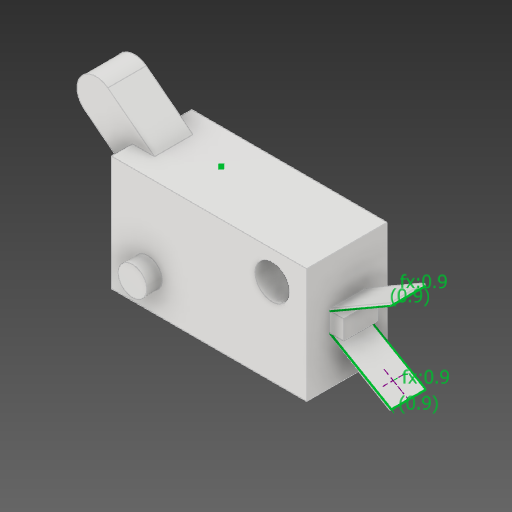
# Autodesk Inventor part: LimitSwitch
Saved by Autodesk Inventor 2019 (Build 230136000, 136)
## iProperties
Created: 2019-04-29
Part Number: LimitSwitch
Material: ABS Plastic
Document SubType Name: Modeling
Designer: skylercleland
Density: 1.06 g/cm^3
Appearance: Smooth - White
Mass: 0.281544 g
Surface Area: 3.43625 cm^2
Volume: 0.265608 cm^3
Name: Limit Switch
Author: skylercleland
Autodesk Inventor part; units mm, degrees
ref_plane "YZ Plane" through (0, 0, 0) normal (1, 0, 0) x (0, 1, 0)
ref_plane "XZ Plane" through (0, 0, 0) normal (0, 1, 0) x (-1, 0, 0)
ref_plane "XY Plane" through (0, 0, 0) normal (0, 0, 1) x (1, 0, 0)
sketch "Sketch1" plane through (0, 0, 0) normal (0, 0, 1) x (1, 0, 0)
  line L0 (0, 0) -> (10.2, 0)
  line L1 (10.2, 0) -> (10.2, 6)
  line L2 (10.2, 6) -> (0, 6)
  line L3 (0, 6) -> (0, 0)
  circle A0 centre (8.4, 4.5) radius 0.9
  line L4 (10.2, 3.5) -> (10.9353, 3.5)
  line L5 (10.9353, 3.5) -> (10.9353, 2.5)
  line L6 (10.9353, 2.5) -> (10.2, 2.5)
  line L7 (10.2, 2.5) -> (10.2, 3.5)
  line L8 (10.2, 3.5) -> (10.15, 3.5866)
  line L9 (10.15, 3.5866) -> (13.35, 5.4341)
  line L10 (13.35, 5.4341) -> (13.4, 5.3475)
  line L11 (13.4, 5.3475) -> (10.2, 3.5)
  line L12 (10.2, 2.5) -> (10.15, 2.4134)
  line L13 (10.15, 2.4134) -> (13.35, 0.5659)
  line L14 (13.35, 0.5659) -> (13.4, 0.6525)
  line L15 (13.4, 0.6525) -> (10.2, 2.5)
  circle A1 centre (1.9, 1.7) radius 0.75
  line L16 (0, 4.3634) -> (-2.5124, 6.3094)
  line L17 (-2.5124, 6.3094) -> (-1.2876, 7.8906)
  line L18 (-1.2876, 7.8906) -> (1.1531, 6)
  arc A2 (-1.2876, 7.8906) -> (-2.5124, 6.3094) centre (-1.9, 7.1) ccw
  point P0 (10.9353, 3)
  point P1 (10.2, 3)
  dimension "d0" = 10.2
  dimension "d1" = 6
  dimension "d2" = 1.8
  dimension "d3" = 1.5
  dimension "d4" = 1.8
  dimension "d5" = 2.8
  dimension "d6" = 6.5
  dimension "d7" = 1.5
  dimension "d8" = 0.1
  dimension "d9" = 0.1
  dimension "d10" = 2.1
  dimension "d11" = 13.1
  dimension "d12" = 30
  dimension "d13" = 30
  dimension "d15" = 1
  dimension "d16" = 5
  dimension "d17" = 2
  constraints: 38 end point, 9 parallel, 5 perpendicular, 3 centre point, 3 midpoint, 3 point on line, 2 horizontal, 2 point on circle, 1 horizontal alignment, 1 vertical alignment
  measures "d0" distance of L2.end L1.end
  measures "d1" distance of L1.end L0.end
  measures "d2" distance from line of L1 A0.centre
  measures "d3" distance from line of L2 A0.centre
  measures "d4" diameter of A0
  measures "d5" vertical distance of A0.centre A1.centre
  measures "d6" horizontal distance of A0.centre A1.centre
  measures "d7" diameter of A1
  measures "d8" distance between parallel lines of L15 L13
  measures "d9" distance between parallel lines of L9 L11
  measures "d12" angle of L15 L6
  measures "d13" angle of L4 L11
  measures "d15" distance between parallel lines of L6 L4
  measures "d16" horizontal distance of A0.centre L10.end
  measures "d17" distance between parallel lines of L16 L18
extrude "Extrusion1" add sketch "Sketch1" along normal mid plane 4.2 contours L3 L2 L1 L9 L8 L12 L13 L0 | L13 L12 L1 | L8 L9 L1
extrude "Extrusion2" add sketch "Sketch1" along normal mid plane 1.8 contours L13 L12 L1 | L1 L15 L14 L13 | L1 L4 L5 L6 | L8 L9 L1 | L1 L9 L10 L11
extrude "Extrusion3" add sketch "Sketch1" along normal mid plane 5.8 contours A1
extrude "Extrusion4" add sketch "Sketch1" along normal mid plane 2 contours L16 L17 L18 L2 L3 | A2 L17
sketch "Sketch2" plane through (10.2, 2.5, 0.9) normal (0.5, 0.866, 0) x (0.866, -0.5, 0)
  line L0 (0, 0) -> (0, 1.8) projected
  line L1 (3.695, 0) -> (0, 0) projected
  line L2 (3.695, 1.8) -> (3.695, 0) projected
  line L3 (0, 1.8) -> (3.695, 1.8) projected
  line L4 (2.795, 0.9) -> (3.695, 0.9) construction
  point P0 (-7.5835, 0.9)
  dimension "d26" = 0.9
  dimension "d27" = 0.9
  constraints: 2 end point, 1 midpoint, 1 perpendicular
  measures "d26" distance between parallel lines of L1 L4
  measures "d27" distance from line of L2 L4.start
sketch "Sketch3" plane through (13.4, 5.3475, -0.9) normal (0.5, -0.866, 0) x (0.866, 0.5, 0)
  line L0 (0, 0) -> (0, 1.8) projected
  line L1 (-3.695, 1.8) -> (0, 1.8) projected
  line L2 (-3.695, 0) -> (-3.695, 1.8) projected
  line L3 (0, 0) -> (-3.695, 0) projected
  line L4 (0, 0) -> (0, 1.8) construction
  line L5 (0, 0.9) -> (-0.9, 0.9) construction
  point P0 (-14.2785, 0.9)
  dimension "d28" = 0.9
  dimension "d29" = 0.9
  constraints: 2 end point, 1 coincident, 1 horizontal, 1 midpoint
  measures "d28" distance between parallel lines of L3 L5
  measures "d29" distance from line of L0 L5.end
equation "\"d27\" = d26"
equation "\"d29\" = d28"
body "Solid1"
